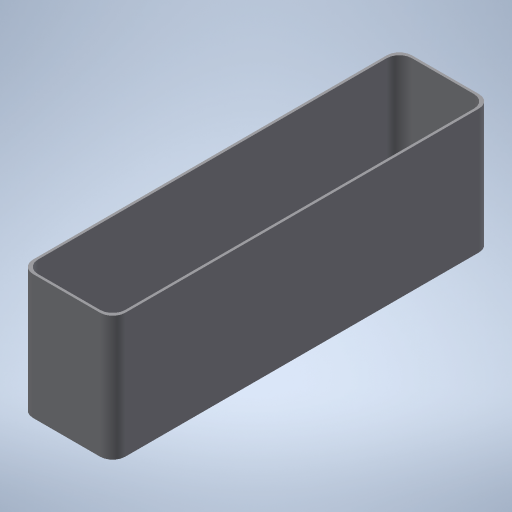
# Autodesk Inventor part: cinta
Saved by Autodesk Inventor 2023 (Build 270158000, 158)
## iProperties
Created: 2022-10-18
Part Number: cinta
Material: Generic
Document SubType Name: Modeling
Designer: Xiaba
Density: 1 g/cm^3
Appearance: Default
Author: Xiaba
Autodesk Inventor part; units mm, degrees
ref_plane "YZ Plane" through (0, 0, 0) normal (1, 0, 0) x (0, 1, 0)
ref_plane "XZ Plane" through (0, 0, 0) normal (0, 1, 0) x (-1, 0, 0)
ref_plane "XY Plane" through (0, 0, 0) normal (0, 0, 1) x (1, 0, 0)
sketch "Sketch1" plane through (0, 0, 0) normal (0, 1, 0) x (-1, 0, 0)
  line L0 (13.796, 28.5881) -> (3.796, 28.5881)
  line L1 (1.796, 26.5881) -> (1.796, -29.4119)
  line L2 (3.796, -31.4119) -> (13.796, -31.4119)
  line L3 (15.796, -29.4119) -> (15.796, 26.5881)
  arc A0 (15.796, 26.5881) -> (13.796, 28.5881) centre (13.796, 26.5881) ccw
  arc A1 (13.796, -31.4119) -> (15.796, -29.4119) centre (13.796, -29.4119) ccw
  arc A2 (1.796, -29.4119) -> (3.796, -31.4119) centre (3.796, -29.4119) ccw
  arc A3 (3.796, 28.5881) -> (1.796, 26.5881) centre (3.796, 26.5881) ccw
  line L4 (14.196, 28.9881) -> (3.396, 28.9881)
  line L5 (1.396, 26.9881) -> (1.396, -29.8119)
  line L6 (3.396, -31.8119) -> (14.196, -31.8119)
  line L7 (16.196, -29.8119) -> (16.196, 26.9881)
  arc A4 (16.196, 26.9881) -> (14.196, 28.9881) centre (14.196, 26.9881) ccw
  arc A5 (14.196, -31.8119) -> (16.196, -29.8119) centre (14.196, -29.8119) ccw
  arc A6 (1.396, -29.8119) -> (3.396, -31.8119) centre (3.396, -29.8119) ccw
  arc A7 (3.396, 28.9881) -> (1.396, 26.9881) centre (3.396, 26.9881) ccw
  point P0 (0, 0)
  point P1 (15.796, 28.5881)
  point P2 (1.796, -31.4119)
  point P3 (15.796, -31.4119)
  dimension "d0" = 60
  dimension "d1" = 14
  dimension "d2" = 2
  dimension "d3" = 0.4
  dimension "d4" = 0.4
  dimension "d5" = 0.4
  dimension "d6" = 0.4
  dimension "d7" = 2
  constraints: 16 end point, 16 point on circle, 16 tangent, 8 centre point, 6 equal radius, 6 point on line, 4 parallel, 2 horizontal, 2 perpendicular
  measures "d0" distance of point (15.796, -31.412) point (15.796, 28.588)
  measures "d1" distance of point (1.796, -31.412) point (15.796, -31.412)
  measures "d2" radius of A0
  measures "d3" distance between parallel lines of L2 L6
  measures "d4" distance between parallel lines of L0 L4
  measures "d5" distance between parallel lines of L3 L7
  measures "d6" distance between parallel lines of L5 L1
  measures "d7" radius of A4
extrude "Extrusion1" add sketch "Sketch1" along normal blind 20
body "Solid1"
